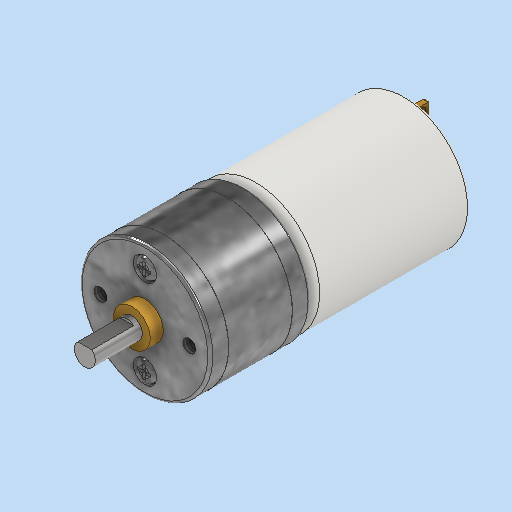
# Autodesk Inventor part: 25ga-370-280-rpm-dc Motor
Saved by Autodesk Inventor 2026 (Build 300175000, 175)
## iProperties
Created: 2021-05-12
Part Number: 25ga-370-280-rpm-dc Motor
Material: Generic
Document SubType Name: Modeling
Designer: Suriyan.S
Density: 1 g/cm^3
Appearance: Titanium - Polished
Author: Suriyan.S
Autodesk Inventor part; units mm, degrees
ref_plane "YZ Plane" through (0, 0, 0) normal (1, 0, 0) x (0, 1, 0)
ref_plane "XZ Plane" through (0, 0, 0) normal (0, 1, 0) x (-1, 0, 0)
ref_plane "XY Plane" through (0, 0, 0) normal (0, 0, 1) x (1, 0, 0)
sketch "Sketch1" plane through (0, 0, 0) normal (0, 0, 1) x (1, 0, 0)
  circle A0 centre (0, 0) radius 12.2
  dimension "d0" = 24.4
  constraints: 1 centre point, 1 coincident
  measures "d0" diameter of A0
extrude "Extrusion1" add sketch "Sketch1" against normal blind 30.8
fillet "Fillet1" radius 2 1 edges at (-12.2, 0, 0)
sketch "Sketch2" plane through (0, 0, 0) normal (1, 0, 0) x (0, 1, 0)
  line L0 (7.5, -26.8) -> (9.5, -26.8)
  line L1 (9.5, -26.8) -> (9.5, -34.8)
  line L2 (9.5, -34.8) -> (7.5, -34.8)
  line L3 (7.5, -34.8) -> (7.5, -26.8)
  line L4 (-12.2, -30.8) -> (12.2, -30.8) construction
  line L5 (7.5, -26.8) -> (9.5, -34.8) construction
  line L6 (9.5, -26.8) -> (7.5, -34.8) construction
  line L7 (-9.5, -26.8) -> (-7.5, -26.8)
  line L8 (-7.5, -26.8) -> (-7.5, -34.8)
  line L9 (-7.5, -34.8) -> (-9.5, -34.8)
  line L10 (-9.5, -34.8) -> (-9.5, -26.8)
  line L11 (-9.5, -26.8) -> (-7.5, -34.8) construction
  line L12 (-7.5, -26.8) -> (-9.5, -34.8) construction
  line L13 (0, 0) -> (0, -39.6837) construction
  circle A0 centre (8.5, -33.3) radius 0.75
  circle A1 centre (-8.5, -33.3) radius 0.75
  line L14 (9.5, -30.8) -> (7.5, -30.8)
  line L15 (-7.5, -30.8) -> (-9.5, -30.8)
  point P0 (8.5, -30.8)
  point P1 (-8.5, -30.8)
  point P2 (8.5, -34.8)
  point P3 (-8.5, -34.8)
  dimension "d4" = 2
  dimension "d5" = 2
  dimension "d6" = 8
  dimension "d7" = 15
  dimension "d8" = 7.5
  dimension "d9" = 1.5
  dimension "d10" = 1.5
  constraints: 30 end point, 10 midpoint, 5 point on line, 4 parallel, 2 centre point, 2 horizontal, 2 perpendicular, 2 vertical alignment, 1 equal radius, 1 horizontal alignment, 1 vertical
  measures "d4" distance of L8.end L9.end
  measures "d5" distance of L1.end L2.end
  measures "d6" distance of L0.end L1.end
  measures "d7" distance between parallel lines of L8 L3
  measures "d8" distance between parallel lines of L3 L13
  measures "d9" distance from line of A0.centre L2
  measures "d10" diameter of A0
extrude "Extrusion2" add sketch "Sketch2" along normal mid plane 1 separate body contours L14 L1 L2 L3 | L15 L8 L9 L10
chamfer "Chamfer1" distance 0.3 angle 45 4 edges at (0.5, 8.5, -34.8) (-0.5, 8.5, -34.8) (0.5, -8.5, -34.8) (-0.5, -8.5, -34.8)
fillet "Fillet3" radius 0.3 4 edges at (0, -7.5, -34.8) (0, -9.5, -34.8) (0, 9.5, -34.8) (0, 7.5, -34.8)
sketch "Sketch3" plane through (0, 0, -30.8) normal (0, 0, -1) x (-1, 0, 0)
  circle A0 centre (0, 0) radius 12.2 construction
  circle A1 centre (0, 0) radius 3.25
  dimension "d18" = 6.5
  constraints: 1 centre point, 1 coincident
  measures "d18" diameter of A1
extrude "Extrusion3" add sketch "Sketch3" along normal blind 2 separate body
fillet "Fillet4" radius 0.5 1 edges at (3.25, 0, -32.8)
sketch "Sketch4" plane through (0, 0, 0) normal (0, 0, 1) x (1, 0, 0)
  circle A0 centre (0, 0) radius 3.25 construction
  circle A1 centre (0, 0) radius 12.5
  dimension "d22" = 25
  constraints: 1 centre point, 1 coincident
  measures "d22" diameter of A1
extrude "Extrusion4" add sketch "Sketch4" along normal blind 19.2 separate body
fillet "Fillet5" radius 0.5 2 edges at (-12.5, 0, 0) (-12.5, 0, 19.2)
sketch "Sketch5" plane through (0, 0, 19.2) normal (0, 0, 1) x (1, 0, 0)
  circle A0 centre (0, 0) radius 3.25 construction
  circle A1 centre (0, 0) radius 3.5
  dimension "d26" = 7
  constraints: 1 centre point, 1 coincident
  measures "d26" diameter of A1
extrude "Extrusion5" add sketch "Sketch5" along normal blind 2.5 separate body
sketch "Sketch6" plane through (0, 0, 21.7) normal (0, 0, 1) x (1, 0, 0)
  circle A0 centre (0, 0) radius 3.25 construction
  circle A1 centre (0, 0) radius 2
  dimension "d29" = 4
  constraints: 1 centre point, 1 coincident
  measures "d29" diameter of A1
extrude "Extrusion6" add sketch "Sketch6" along normal blind 9 separate body
sketch "Sketch7" plane through (0, 0, 30.7) normal (0, 0, 1) x (1, 0, 0)
  circle A0 centre (0, 0) radius 2 projected
  line L0 (-2.5, 1.5) -> (2.5, 1.5)
  line L1 (2.5, 1.5) -> (2.5, -1.5)
  line L2 (2.5, -1.5) -> (-2.5, -1.5)
  line L3 (-2.5, -1.5) -> (-2.5, 1.5)
  line L4 (-2.5, 1.5) -> (2.5, -1.5) construction
  line L5 (2.5, 1.5) -> (-2.5, -1.5) construction
  point P0 (-1.3229, 1.5)
  point P1 (1.3229, 1.5)
  dimension "d32" = 1.5
  dimension "d33" = 5
  constraints: 12 end point, 2 midpoint, 2 parallel, 1 horizontal, 1 perpendicular
  measures "d32" distance from line of A0.centre L0
  measures "d33" distance of L1.end L2.end
extrude "Extrusion7" cut sketch "Sketch7" against normal blind 8 contours L0 A0 bodies 6
sketch "Sketch8" plane through (0, 0, 0) normal (1, 0, 0) x (0, 1, 0)
  line L0 (12.75, 15.71) -> (12.25, 15.71)
  line L1 (12.25, 15.71) -> (12.25, 15.69)
  line L2 (12.25, 15.69) -> (12.75, 15.69)
  line L3 (12.75, 15.69) -> (12.75, 15.71)
  line L4 (12.5, 0.5) -> (12.5, 18.7) construction
  line L5 (12.75, 15.71) -> (12.25, 15.69) construction
  line L6 (12.25, 15.71) -> (12.75, 15.69) construction
  line L7 (12.75, 3.49) -> (12.25, 3.49)
  line L8 (12.25, 3.49) -> (12.25, 3.51)
  line L9 (12.25, 3.51) -> (12.75, 3.51)
  line L10 (12.75, 3.51) -> (12.75, 3.49)
  line L11 (12.75, 3.49) -> (12.25, 3.51) construction
  line L12 (12.25, 3.49) -> (12.75, 3.51) construction
  line L13 (-12, 19.2) -> (12, 19.2) construction
  line L14 (12, 0) -> (-12, 0) construction
  line L15 (0, -3.84) -> (0, 23.04) projected
  point P0 (0, 0)
  point P1 (12.5, 15.7)
  point P2 (12.5, 3.5)
  dimension "d36" = 0.02
  dimension "d37" = 0.5
  dimension "d38" = 3.5
  dimension "d39" = 3.5
  constraints: 24 end point, 4 midpoint, 4 parallel, 3 point on line, 2 horizontal, 2 perpendicular, 1 collinear
  measures "d36" distance of L2.end L0.start
  measures "d37" distance of L1.end L2.end
  measures "d38" distance from line of L13 point (12.5, 15.7)
  measures "d39" distance from line of L14 point (12.5, 3.5)
revolve "Revolution1" cut sketch "Sketch8" angle 360 about axis through (0, 0, -10) along (0, 0, 1) bodies 4
fillet "Fillet6" radius 0.01 1 edges at (-12.5, 0, 15.69)
fillet "Fillet7" radius 0.01 1 edges at (-12.5, 0, 3.51)
sketch "Sketch9" plane through (0, 0, 19.2) normal (0, 0, 1) x (1, 0, 0)
  point P0 (0, 0)
  point P1 (0, 8.5)
  point P2 (0, -8.5)
  dimension "d50" = 17
  dimension "d51" = 8.5
  constraints: 2 vertical alignment
  measures "d50" distance of point (0, -8.5) point (0, 8.5)
  measures "d51" distance of point (0, -8.5) point (0, 0)
hole "Hole1" at (0, 8.5, 19.2) at (0, -8.5, 19.2) direction (0, 0, -1) diameter 2.4 depth 8 tip angle 118 counterbore diameter 4.4 counterbore depth 2.3 bodies 4 clearance for "Socket Head Cap Screw ISO 4762" size "M2" standard "ISO"
sketch "Sketch10" plane through (0, 0, 19.2) normal (0, 0, 1) x (1, 0, 0)
  circle A0 centre (0, 0) radius 3.25 construction
  circle A1 centre (0, 0) radius 8.5
  point P0 (8.5, 0)
  point P1 (-8.5, 0)
  dimension "d59" = 17
  constraints: 2 horizontal alignment, 2 point on circle, 1 centre point, 1 coincident
  measures "d59" diameter of A1
hole "Hole2" at (8.5, 0, 19.2) at (-8.5, 0, 19.2) direction (0, 0, -1) diameter 2.459 depth 8.8 tip angle 118 bodies 4 thread size "M3x0.5" class "6H" standard "ISO Metric profile"
sketch "Sketch11" plane through (0, 8.5, 16.9) normal (0, 0, 1) x (1, 0, 0)
  circle A0 centre (0, 0) radius 1.2 construction
  circle A1 centre (0, 0) radius 2
  point P0 (0, -8.5)
  dimension "d60" = 4
  constraints: 1 centre point
  measures "d60" diameter of A1
extrude "Extrusion8" add sketch "Sketch11" along normal blind 2.5 bodies 4
fillet "Fillet8" radius 1 1 edges at (-2, 8.5, 19.4)
sketch "Sketch12" plane through (0, 8.5, 19.4) normal (0, 0, 1) x (1, 0, 0)
  circle A0 centre (0, 0) radius 1 construction
  line L0 (-1.25, 0.25) -> (1.25, 0.25)
  line L1 (1.25, 0.25) -> (1.25, -0.25)
  line L2 (1.25, -0.25) -> (-1.25, -0.25)
  line L3 (-1.25, -0.25) -> (-1.25, 0.25)
  line L4 (-1.25, 0.25) -> (1.25, -0.25) construction
  line L5 (1.25, 0.25) -> (-1.25, -0.25) construction
  line L6 (-0.25, 1.25) -> (0.25, 1.25)
  line L7 (0.25, 1.25) -> (0.25, -1.25)
  line L8 (0.25, -1.25) -> (-0.25, -1.25)
  line L9 (-0.25, -1.25) -> (-0.25, 1.25)
  line L10 (-0.25, 1.25) -> (0.25, -1.25) construction
  line L11 (0.25, 1.25) -> (-0.25, -1.25) construction
  point P0 (0, -8.5)
  point P1 (-0.25, 0.25)
  point P2 (-0.25, -0.25)
  point P3 (0.25, -0.25)
  point P4 (0.25, 0.25)
  dimension "d64" = 2.5
  dimension "d65" = 0.5
  dimension "d66" = 0.5
  constraints: 24 end point, 4 midpoint, 4 parallel, 3 perpendicular, 2 horizontal
  measures "d64" distance of L6.end L7.end
  measures "d65" distance of L6.start L6.end
  measures "d66" distance of L0.end L1.end
extrude "Extrusion9" cut sketch "Sketch12" against normal blind 0.5 bodies 4
pattern_circular "Circular Pattern1" count 2 over 360 about axis through (0, 0, 0) along (0, 0, 1) of "Extrusion9", "Fillet8", "Extrusion8" bodies 4
fillet "Fillet9" radius 0.5 1 edges at (-12.2, 0, -30.8)
equation "\"d5\" = d4"
equation "\"d8\" = 0.5 * d7"
equation "\"d51\" = 0.5 * d50"
equation "\"d38\" = d39"
body "Solid1"
body "Solid2"
body "Solid3"
body "Solid4"
body "Solid5"
body "Solid6"
